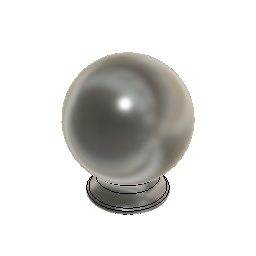
Joystick_sfera_rev_1.0 (Autodesk Fusion 360 design; units mm, degrees)
Autodesk Fusion 360 part; units mm, degrees
sketch "Schizzo1" plane through (0, 0, 0) normal (1, 0, 0) x (0, 1, 0)
  line L0 (0, 0) -> (3.225, 0) construction
  line L1 (20.0798, -7.3107) -> (21.2628, -8.3935)
  line L2 (3.225, 15) -> (0, 15)
  arc A0 (17, 5) -> (20.0798, -7.3107) centre (27.8443, 1.1723) ccw
  line L3 (20.25, -11) -> (20.25, -9.5) construction
  arc A1 (20.25, -11) -> (21.2628, -8.3935) centre (20.25, -9.5) ccw
  line L4 (3.225, 0) -> (3.225, 15)
  line L5 (20.25, -9.5) -> (21.75, -9.5) construction
  line L6 (3.225, 0) -> (17.033, -10.788)
  line L7 (20.25, -11) -> (17.6487, -11)
  arc A2 (17.033, -10.788) -> (17.6487, -11) centre (17.6487, -10) ccw
  line L8 (0, 0) -> (0, 15) construction
  line L9 (0, 15) -> (0, 34.7908)
  line L10 (0, 34.7908) -> (0, 69.0908)
  arc A3 (17, 5) -> (0, 69.0908) centre (0, 34.7908) ccw
  point P0 (11, 1)
  dimension "d1" = 3.225
  dimension "d2" = 15
  dimension "d6" = 3
  dimension "d7" = 21.75
  dimension "d8" = 11
  dimension "d9" = 1
  dimension "d24" = 11.5
  dimension "d41" = 4
  dimension "d48" = 1
  dimension "d49" = 142
  dimension "d50" = 11
  dimension "d22" = 68.6
  dimension "d23" = 17
  constraint vertical L4
  constraint perpendicular L2 L4
  constraint coincident L0.start L8.start
  constraint perpendicular L2 L8
  constraint perpendicular L0 L4
  constraint coincident L3.start A1.start
  constraint coincident L3.end A1.centre
  constraint vertical L3
  constraint coincident L5.end A1
  constraint perpendicular L3 L5
  constraint tangent L1 A1
  constraint coincident P0 L1
  constraint tangent L1 A0
  constraint tangent L6 A2
  constraint tangent L7 A2
  constraint coincident L9.end L10.start
  constraint vertical L9
  constraint parallel L9 L10
  measures "d1" distance of L4 L8
  measures "d2" distance of L2.start L0.end
  measures "d6" diameter of A1
  measures "d7" distance of L5.end L8
  measures "d8" distance of P0 L8
  measures "d9" vertical distance of P0 L0.end
  measures "d24" radius of A0
  measures "d41" vertical distance of P0 A0.start
  measures "d48" radius of A2
  measures "d49" angle of L6 L7
  measures "d50" distance of L0 L7
  measures "d22" diameter of A3
  measures "d23" distance of A0.start L8
revolve "Rivoluzione1" add sketch "Schizzo1" angle 360 about axis through (0, 0, 0) along (0, 0, 1)
fillet "Raccordo1" radius 7.4973 1 edges at (-15.8496, 6.1475, 5)
equation "d1 = larghezza_incastro_joystick / 2"
equation "d7 = ( 43.5 / 2 ) * 1 mm"
equation "d8 = ( 22 / 2 ) * 1 mm"
equation "diametro_sfera_joystick = 68.6 mm" comment "Modificare questo valore per aumentare o diminuire il diametro della sfera del joystick. (Valore di default 68.6 mm)"
equation "larghezza_incastro_joystick = 6.45 mm" comment "Modificare questo valore per allargare o diminuire il foro dell'incastro del Joystick. (Valore di default 6.45 mm)"
equation "d22 = diametro_sfera_joystick"
equation "d27 = diametro_sfera_joystick / 9.15"
named bodies: "joystick_sfera"
